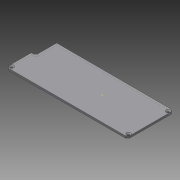
# Autodesk Inventor part: main body cover
Saved by Autodesk Inventor 2015 (Build 190159000, 159)
## iProperties
Created: 2019-05-11
Part Number: main body cover
Material: Generic
Document SubType Name: Modeling
Designer: Toby
Density: 1 g/cm^3
Appearance: Default
Author: Toby
Autodesk Inventor part; units mm, degrees
ref_plane "YZ Plane" through (0, 0, 0) normal (1, 0, 0) x (0, 1, 0)
ref_plane "XZ Plane" through (0, 0, 0) normal (0, 1, 0) x (-1, 0, 0)
ref_plane "XY Plane" through (0, 0, 0) normal (0, 0, 1) x (1, 0, 0)
sketch "Sketch1" plane through (0, 0, 0) normal (1, 0, 0) x (0, 1, 0)
  point P0 (0, 0)
sketch "Sketch2" plane through (0, 0, 0) normal (0, 0, 1) x (1, 0, 0)
  line L0 (-65.94, 18.9) -> (48.46, 18.9)
  line L1 (48.46, 18.9) -> (48.46, -24.5)
  line L2 (48.46, -24.5) -> (-65.94, -24.5)
  line L3 (-65.94, -24.5) -> (-65.94, 18.9)
  point P0 (0, 0)
  dimension "d0" = 43.4
  dimension "d1" = 114.4
  constraints: 8 end point, 2 parallel, 1 horizontal, 1 perpendicular
  measures "d0" distance between parallel lines of L2 L0
  measures "d1" distance between parallel lines of L1 L3
extrude "Extrusion1" add sketch "Sketch2" along normal blind 2
chamfer "Chamfer1" distance 2 angle 45 3 edges at (48.46, 18.9, 1) (48.46, -24.5, 1) (-65.94, -24.5, 1)
sketch "Sketch3" plane through (0, 0, 2) normal (0, 0, 1) x (1, 0, 0)
  line L0 (-65.94, 18.9) -> (-61.94, 18.9)
  line L1 (-61.94, 18.9) -> (-61.94, -1.1)
  line L2 (-61.94, -1.1) -> (-65.94, -1.1)
  line L3 (-65.94, -1.1) -> (-65.94, 18.9)
  point P0 (0, 0)
  dimension "d7" = 4
  dimension "d8" = 20
  constraints: 8 end point, 2 parallel, 1 horizontal, 1 perpendicular
  measures "d7" distance of L1.end L2.end
  measures "d8" distance of L0.end L1.end
extrude "Extrusion2" cut sketch "Sketch3" against normal blind 2
chamfer "Chamfer2" distance 2 angle 45 1 edges at (-61.94, -1.1, 1)
sketch "Sketch4" plane through (0, 0, 2) normal (0, 0, 1) x (1, 0, 0)
  line L0 (-61.94, 18.9) -> (46.46, 18.9) projected
  line L1 (-63.94, -24.5) -> (46.46, -24.5) projected
  line L2 (48.46, -22.5) -> (48.46, 16.9) projected
  line L3 (-65.94, -22.5) -> (-65.94, -1.1) projected
  point P0 (0, 0)
  point P1 (-63.94, -21.5)
  point P2 (46.46, -21.5)
  point P3 (46.46, 15.9)
  dimension "d14" = 3
  dimension "d15" = 3
  dimension "d16" = 2
  dimension "d17" = 2
  dimension "d18" = 2
  dimension "d19" = 3
  measures "d14" distance from line of L0 point (46.46, 15.9)
  measures "d15" distance from line of L1 point (46.46, -21.5)
  measures "d16" distance from line of L2 point (46.46, 15.9)
  measures "d17" distance from line of L2 point (46.46, -21.5)
  measures "d18" distance from line of L3 point (-63.94, -21.5)
  measures "d19" distance from line of L1 point (-63.94, -21.5)
hole "Hole1" at (-63.94, -21.5, 2) at (46.46, -21.5, 2) at (46.46, 15.9, 2) direction (0, 0, -1) diameter 2 depth 8 tip angle 118 countersink diameter 4 countersink angle 90
body "Solid1"
